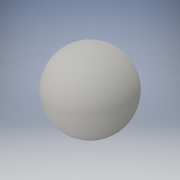
# Autodesk Inventor part: Sphere
Saved by Autodesk Inventor 2016 (Build 200138000, 138)
## iProperties
Created: 2017-10-18
Part Number: Sphere
Material: Generic
Document SubType Name: Modeling
Designer: ls769
Density: 1 g/cm^3
Appearance: Default
Author: ls769
Autodesk Inventor part; units mm, degrees
ref_plane "YZ Plane" through (0, 0, 0) normal (1, 0, 0) x (0, 1, 0)
ref_plane "XZ Plane" through (0, 0, 0) normal (0, 1, 0) x (-1, 0, 0)
ref_plane "XY Plane" through (0, 0, 0) normal (0, 0, 1) x (1, 0, 0)
sketch "Sketch3" plane through (0, 0, 0) normal (0, 0, 1) x (1, 0, 0)
  arc A0 (0, -15) -> (0, 15) centre (0, 0) ccw
  arc A1 (0, -9) -> (0, 9) centre (0, 0) ccw
  line L0 (0, 16.0559) -> (0, 15)
  line L1 (0, 15) -> (0, -9)
  line L2 (0, -9) -> (0, -15)
  line L3 (0, -15) -> (0, -17.0253)
  line L4 (0, -23.6415) -> (0, 22.6721) projected
  dimension "d4" = 30
  dimension "d5" = 18
  constraints: 8 end point, 4 point on circle, 4 vertical, 3 point on line, 2 centre point, 2 coincident
  measures "d4" diameter of A0
  measures "d5" diameter of A1
revolve "Revolution2" add sketch "Sketch3" angle 360 about axis through (0, -10, 0) along (0, 1, 0) contours L2 A1 L1 A0
body "Solid2"
